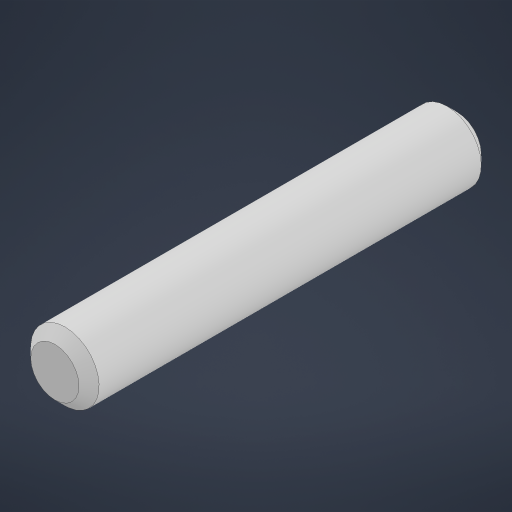
# Autodesk Inventor part: Axle Small
Saved by Autodesk Inventor 2023.2 (Build 272271000, 271)
## iProperties
Created: 2022-11-29
Part Number: Axle Small
Material: Generic
Document SubType Name: Modeling
Designer: iusti
Density: 1 g/cm^3
Appearance: Gunmetal - Antique Polished
Author: iusti
Autodesk Inventor part; units mm, degrees
ref_plane "YZ Plane" through (0, 0, 0) normal (1, 0, 0) x (0, 1, 0)
ref_plane "XZ Plane" through (0, 0, 0) normal (0, 1, 0) x (-1, 0, 0)
ref_plane "XY Plane" through (0, 0, 0) normal (0, 0, 1) x (1, 0, 0)
sketch "Sketch1" plane through (0, 0, 0) normal (1, 0, 0) x (0, 1, 0)
  line L0 (1.7, 10) -> (0, 10)
  line L1 (0, 10) -> (0, -10)
  line L2 (0, -10) -> (1.7, -10)
  line L3 (1.7, -10) -> (1.7, 10)
  point P0 (0, 0)
  point P1 (0, 0)
  dimension "d0" = 20
  dimension "d1" = 3.4
  constraints: 8 end point, 2 parallel, 1 coincident, 1 horizontal, 1 midpoint, 1 perpendicular
  measures "d0" distance of L2.end L0.start
  measures "d1" diameter of L3 L1
revolve "Revolution1" add sketch "Sketch1" angle 360 about axis through (0, 0, 10) along (0, 0, -1)
chamfer "Chamfer1" distance 0.5 angle 45 2 edges at (0, -1.7, 10) (0, -1.7, -10)
body "Solid1"
